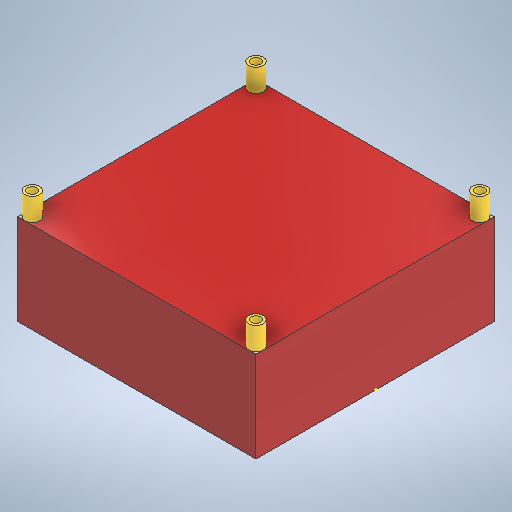
# Autodesk Inventor part: Sensor_Release_Magnet
Saved by Autodesk Inventor 2025.1 (Build 291241020, 241B)
## iProperties
Created: 2025-02-15
Part Number: Sensor_Release_Magnet
Material: Generic
Document SubType Name: Modeling
Designer: smyth
Density: 1 g/cm^3
Appearance: Default
Author: smyth
Autodesk Inventor part; units mm, degrees
ref_plane "YZ Plane" through (0, 0, 0) normal (1, 0, 0) x (0, 1, 0)
ref_plane "XZ Plane" through (0, 0, 0) normal (0, 1, 0) x (-1, 0, 0)
ref_plane "XY Plane" through (0, 0, 0) normal (0, 0, 1) x (1, 0, 0)
sketch "Sketch1" plane through (0, 0, 0) normal (0, 1, 0) x (-1, 0, 0)
  line L0 (-18.669, 18.669) -> (18.669, 18.669)
  line L1 (18.669, 18.669) -> (18.669, -18.669)
  line L2 (18.669, -18.669) -> (-18.669, -18.669)
  line L3 (-18.669, -18.669) -> (-18.669, 18.669)
  line L4 (-18.669, 18.669) -> (18.669, -18.669) construction
  line L5 (18.669, 18.669) -> (-18.669, -18.669) construction
  point P0 (0, 0)
  dimension "d0" = 37.338
  constraints: 12 end point, 2 midpoint, 2 parallel, 1 horizontal, 1 perpendicular
  measures "d0" distance of L0.end L1.end
extrude "Extrusion1" add sketch "Sketch1" along normal blind 14.224
sketch "Sketch2" plane through (18.669, 0, 18.669) normal (1, 0, 0) x (0, 0, -1)
  point P0 (18.669, 0)
sketch "Sketch3" plane through (0, 14.224, 0) normal (0, 1, 0) x (1, 0, 0)
  circle A0 centre (-17.526, -17.526) radius 1.143
  line L0 (-18.669, 18.669) -> (-18.669, -18.669) projected
  line L1 (-18.669, -18.669) -> (18.669, -18.669) projected
  circle A1 centre (-17.526, 17.526) radius 1.143
  circle A2 centre (17.526, 17.526) radius 1.143
  circle A3 centre (17.526, -17.526) radius 1.143
  line L2 (18.669, 18.669) -> (-18.669, 18.669) projected
  line L3 (18.669, -18.669) -> (18.669, 18.669) projected
  point P0 (0, 0)
  dimension "d3" = 2.286
  dimension "d4" = 2.286
  dimension "d5" = 2.286
  dimension "d6" = 2.286
  constraints: 8 tangent, 4 centre point
  measures "d3" diameter of A0
  measures "d4" diameter of A3
  measures "d5" diameter of A2
  measures "d6" diameter of A1
extrude "Extrusion2" add sketch "Sketch3" along normal blind 3.556 contours A0 | A1 | A3 | A2
sketch "Sketch4" plane through (-17.526, 17.78, 17.526) normal (0, 1, 0) x (1, 0, 0)
  circle A0 centre (0, 0) radius 0.75
  circle A1 centre (35.052, 0) radius 0.75
  circle A2 centre (35.052, 35.052) radius 0.75
  circle A3 centre (0, 35.052) radius 0.75
  point P0 (17.526, 17.526)
  dimension "d9" = 1.5
  dimension "d10" = 1.5
  dimension "d11" = 1.5
  dimension "d12" = 1.5
  constraints: 4 centre point
  measures "d9" diameter of A0
  measures "d10" diameter of A1
  measures "d11" diameter of A2
  measures "d12" diameter of A3
extrude "Extrusion3" cut sketch "Sketch4" against normal blind 3.556
body "Solid1"
